Autodesk Fusion 360 part; units mm, degrees
(part 2 of 3)
extrude "Extrude4'''''''''" add sketch "Sketch4 (10)" along normal blind 20 separate body contours L0 L1 L2 L3 in plane through (0, 0, 580) normal (0, 0, 1) makes body 111 in component "02_VisionStation (1)"
sketch "Sketch5 (9)" plane through (0, 0, 0) normal (0, 0, 1) x (1, 0, 0) in component "02_VisionStation (1)"
  line L0 (965, 160, 540) -> (1015, 160, 540)
  line L1 (1015, 160, 540) -> (1015, 240, 540)
  line L2 (1015, 240, 540) -> (965, 240, 540)
  line L3 (965, 240, 540) -> (965, 160, 540)
extrude "Extrude5''''''''" add sketch "Sketch5 (9)" along normal blind 40 separate body contours L0 L1 L2 L3 in plane through (0, 0, 540) normal (0, 0, 1) makes body 112 in component "02_VisionStation (1)"
sketch "Sketch6 (9)" plane through (0, 0, 0) normal (0, 0, 1) x (1, 0, 0) in component "02_VisionStation (1)"
  circle A0 through (1002, 200, 520) (984, 210.3923, 520) (984, 189.6077, 520)
extrude "Extrude6''''''''" add sketch "Sketch6 (9)" along normal blind 20 separate body contours A0 in plane through (0, 0, 520) normal (0, 0, 1) makes body 113 in component "02_VisionStation (1)"
sketch "Sketch7 (9)" plane through (0, 0, 0) normal (0, 0, 1) x (1, 0, 0) in component "02_VisionStation (1)"
  line L0 (940, 180, 490) -> (1040, 180, 490)
  line L1 (1040, 180, 490) -> (1040, 220, 490)
  line L2 (1040, 220, 490) -> (940, 220, 490)
  line L3 (940, 220, 490) -> (940, 180, 490)
extrude "Extrude7''''''''" add sketch "Sketch7 (9)" along normal blind 25 separate body contours L0 L1 L2 L3 in plane through (0, 0, 490) normal (0, 0, 1) makes body 114 in component "02_VisionStation (1)"
sketch "Sketch8 (9)" plane through (0, 0, 0) normal (0, 0, 1) x (1, 0, 0) in component "02_VisionStation (1)"
  circle A0 through (972, 195, 480) (961.5, 201.0622, 480) (961.5, 188.9378, 480)
extrude "Extrude8''''''''" add sketch "Sketch8 (9)" along normal blind 10 separate body contours A0 in plane through (0, 0, 480) normal (0, 0, 1) makes body 115 in component "02_VisionStation (1)"
sketch "Sketch9 (9)" plane through (0, 0, 0) normal (0, 0, 1) x (1, 0, 0) in component "02_VisionStation (1)"
  circle A0 through (1022, 195, 480) (1011.5, 201.0622, 480) (1011.5, 188.9378, 480)
extrude "Extrude9''''''''" add sketch "Sketch9 (9)" along normal blind 10 separate body contours A0 in plane through (0, 0, 480) normal (0, 0, 1) makes body 116 in component "02_VisionStation (1)"
sketch "Sketch10 (9)" plane through (0, 0, 0) normal (0, 0, 1) x (1, 0, 0) in component "02_VisionStation (1)"
  circle A0 through (1025, 200, 530) (972.5, 230.3109, 530) (972.5, 169.6891, 530)
extrude "Extrude10''''''''" add sketch "Sketch10 (9)" along normal blind 5 separate body contours A0 in plane through (0, 0, 530) normal (0, 0, 1) makes body 117 in component "02_VisionStation (1)"
sketch "Sketch1 (12)" plane through (0, 0, 0) normal (0, 0, 1) x (1, 0, 0) in component "03_RobotBase (1)"
  line L0 (-200, -200) -> (200, -200)
  line L1 (200, -200) -> (200, 200)
  line L2 (200, 200) -> (-200, 200)
  line L3 (-200, 200) -> (-200, -200)
extrude "Extrude1'''''''''''" add sketch "Sketch1 (12)" along normal blind 30 separate body makes body 118 in component "03_RobotBase (1)"
sketch "Sketch2 (12)" plane through (0, 0, 0) normal (0, 0, 1) x (1, 0, 0) in component "03_RobotBase (1)"
  circle A0 through (150, 0, 30) (-75, 129.9038, 30) (-75, -129.9038, 30)
extrude "Extrude2'''''''''''" add sketch "Sketch2 (12)" along normal blind 100 separate body contours A0 in plane through (0, 0, 30) normal (0, 0, 1) makes body 119 in component "03_RobotBase (1)"
sketch "Sketch3 (11)" plane through (0, 0, 0) normal (0, 0, 1) x (1, 0, 0) in component "03_RobotBase (1)"
  circle A0 through (120, 0, 130) (-60, 103.923, 130) (-60, -103.923, 130)
extrude "Extrude3''''''''''" add sketch "Sketch3 (11)" along normal blind 20 separate body contours A0 in plane through (0, 0, 130) normal (0, 0, 1) makes body 120 in component "03_RobotBase (1)"
sketch "Sketch4 (11)" plane through (0, 0, 0) normal (0, 0, 1) x (1, 0, 0) in component "03_RobotBase (1)"
  line L0 (80, -40, 50) -> (136, -40, 50)
  line L1 (136, -40, 50) -> (136, 16, 50)
  line L2 (136, 16, 50) -> (80, 16, 50)
  line L3 (80, 16, 50) -> (80, -40, 50)
extrude "Extrude4''''''''''" add sketch "Sketch4 (11)" along normal blind 76 separate body contours L0 L1 L2 L3 in plane through (0, 0, 50) normal (0, 0, 1) makes body 121 in component "03_RobotBase (1)"
sketch "Sketch1 (13)" plane through (0, 0, 0) normal (0, 0, 1) x (1, 0, 0) in component "04_RobotArm (1)"
  circle A0 through (80, 0, 150) (-40, 69.282, 150) (-40, -69.282, 150)
extrude "Extrude1''''''''''''" add sketch "Sketch1 (13)" along normal blind 40 separate body contours A0 in plane through (0, 0, 150) normal (0, 0, 1) makes body 122 in component "04_RobotArm (1)"
sketch "Sketch2 (13)" plane through (0, 0, 0) normal (0, 0, 1) x (1, 0, 0) in component "04_RobotArm (1)"
  line L0 (-45, 50, 120) -> (11, 50, 120)
  line L1 (11, 50, 120) -> (11, 106, 120)
  line L2 (11, 106, 120) -> (-45, 106, 120)
  line L3 (-45, 106, 120) -> (-45, 50, 120)
extrude "Extrude2''''''''''''" add sketch "Sketch2 (13)" along normal blind 76 separate body contours L0 L1 L2 L3 in plane through (0, 0, 120) normal (0, 0, 1) makes body 123 in component "04_RobotArm (1)"
sketch "Sketch3 (12)" plane through (0, 0, 0) normal (0, 0, 1) x (1, 0, 0) in component "04_RobotArm (1)"
  line L0 (-20, -20, 190) -> (20, -20, 190)
  line L1 (20, -20, 190) -> (20, 20, 190)
  line L2 (20, 20, 190) -> (-20, 20, 190)
  line L3 (-20, 20, 190) -> (-20, -20, 190)
extrude "Extrude3'''''''''''" add sketch "Sketch3 (12)" along normal blind 400 separate body contours L0 L1 L2 L3 in plane through (0, 0, 190) normal (0, 0, 1) makes body 124 in component "04_RobotArm (1)"
sketch "Sketch4 (12)" plane through (0, 0, 0) normal (0, 0, 1) x (1, 0, 0) in component "04_RobotArm (1)"
  line L0 (-25, -25, 250) -> (25, -25, 250)
  line L1 (25, -25, 250) -> (25, 25, 250)
  line L2 (25, 25, 250) -> (-25, 25, 250)
  line L3 (-25, 25, 250) -> (-25, -25, 250)
extrude "Extrude4'''''''''''" add sketch "Sketch4 (12)" along normal blind 5 separate body contours L0 L1 L2 L3 in plane through (0, 0, 250) normal (0, 0, 1) makes body 125 in component "04_RobotArm (1)"
sketch "Sketch5 (10)" plane through (0, 0, 0) normal (0, 0, 1) x (1, 0, 0) in component "04_RobotArm (1)"
  line L0 (-25, -25, 350) -> (25, -25, 350)
  line L1 (25, -25, 350) -> (25, 25, 350)
  line L2 (25, 25, 350) -> (-25, 25, 350)
  line L3 (-25, 25, 350) -> (-25, -25, 350)
extrude "Extrude5'''''''''" add sketch "Sketch5 (10)" along normal blind 5 separate body contours L0 L1 L2 L3 in plane through (0, 0, 350) normal (0, 0, 1) makes body 126 in component "04_RobotArm (1)"
sketch "Sketch6 (10)" plane through (0, 0, 0) normal (0, 0, 1) x (1, 0, 0) in component "04_RobotArm (1)"
  line L0 (-25, -25, 450) -> (25, -25, 450)
  line L1 (25, -25, 450) -> (25, 25, 450)
  line L2 (25, 25, 450) -> (-25, 25, 450)
  line L3 (-25, 25, 450) -> (-25, -25, 450)
extrude "Extrude6'''''''''" add sketch "Sketch6 (10)" along normal blind 5 separate body contours L0 L1 L2 L3 in plane through (0, 0, 450) normal (0, 0, 1) makes body 127 in component "04_RobotArm (1)"
sketch "Sketch7 (10)" plane through (0, 0, 0) normal (0, 0, 1) x (1, 0, 0) in component "04_RobotArm (1)"
  circle A0 through (60, 0, 590) (-30, 51.9615, 590) (-30, -51.9615, 590)
extrude "Extrude7'''''''''" add sketch "Sketch7 (10)" along normal blind 40 separate body contours A0 in plane through (0, 0, 590) normal (0, 0, 1) makes body 128 in component "04_RobotArm (1)"
sketch "Sketch8 (10)" plane through (0, 0, 0) normal (0, 0, 1) x (1, 0, 0) in component "04_RobotArm (1)"
  line L0 (50, -30, 570) -> (106, -30, 570)
  line L1 (106, -30, 570) -> (106, 26, 570)
  line L2 (106, 26, 570) -> (50, 26, 570)
  line L3 (50, 26, 570) -> (50, -30, 570)
extrude "Extrude8'''''''''" add sketch "Sketch8 (10)" along normal blind 76 separate body contours L0 L1 L2 L3 in plane through (0, 0, 570) normal (0, 0, 1) makes body 129 in component "04_RobotArm (1)"
sketch "Sketch9 (10)" plane through (0, 0, 0) normal (0, 0, 1) x (1, 0, 0) in component "04_RobotArm (1)"
  line L0 (-20, -20, 630) -> (20, -20, 630)
  line L1 (20, -20, 630) -> (20, 20, 630)
  line L2 (20, 20, 630) -> (-20, 20, 630)
  line L3 (-20, 20, 630) -> (-20, -20, 630)
extrude "Extrude9'''''''''" add sketch "Sketch9 (10)" along normal blind 350 separate body contours L0 L1 L2 L3 in plane through (0, 0, 630) normal (0, 0, 1) makes body 130 in component "04_RobotArm (1)"
sketch "Sketch10 (10)" plane through (0, 0, 0) normal (0, 0, 1) x (1, 0, 0) in component "04_RobotArm (1)"
  circle A0 through (50, 0, 980) (-25, 43.3013, 980) (-25, -43.3013, 980)
extrude "Extrude10'''''''''" add sketch "Sketch10 (10)" along normal blind 30 separate body contours A0 in plane through (0, 0, 980) normal (0, 0, 1) makes body 131 in component "04_RobotArm (1)"
sketch "Sketch11 (5)" plane through (0, 0, 0) normal (0, 0, 1) x (1, 0, 0) in component "04_RobotArm (1)"
  line L0 (30, -20, 960) -> (70, -20, 960)
  line L1 (70, -20, 960) -> (70, 20, 960)
  line L2 (70, 20, 960) -> (30, 20, 960)
  line L3 (30, 20, 960) -> (30, -20, 960)
extrude "Extrude11''''" add sketch "Sketch11 (5)" along normal blind 50 separate body contours L0 L1 L2 L3 in plane through (0, 0, 960) normal (0, 0, 1) makes body 132 in component "04_RobotArm (1)"
sketch "Sketch12 (4)" plane through (0, 0, 0) normal (0, 0, 1) x (1, 0, 0) in component "04_RobotArm (1)"
  circle A0 through (-15, 30, 130) (-37.5, 42.9904, 130) (-37.5, 17.0096, 130)
extrude "Extrude12'''" add sketch "Sketch12 (4)" along normal blind 15 separate body contours A0 in plane through (0, 0, 130) normal (0, 0, 1) makes body 133 in component "04_RobotArm (1)"
sketch "Sketch13 (4)" plane through (0, 0, 0) normal (0, 0, 1) x (1, 0, 0) in component "04_RobotArm (1)"
  circle A0 through (-15, 30, 570) (-37.5, 42.9904, 570) (-37.5, 17.0096, 570)
extrude "Extrude13'''" add sketch "Sketch13 (4)" along normal blind 15 separate body contours A0 in plane through (0, 0, 570) normal (0, 0, 1) makes body 134 in component "04_RobotArm (1)"
sketch "Sketch14 (4)" plane through (0, 0, 0) normal (0, 0, 1) x (1, 0, 0) in component "04_RobotArm (1)"
  circle A0 through (-15, 30, 960) (-37.5, 42.9904, 960) (-37.5, 17.0096, 960)
extrude "Extrude14'''" add sketch "Sketch14 (4)" along normal blind 15 separate body contours A0 in plane through (0, 0, 960) normal (0, 0, 1) makes body 135 in component "04_RobotArm (1)"
sketch "Sketch1 (14)" plane through (0, 0, 0) normal (0, 0, 1) x (1, 0, 0) in component "05_Gripper (1)"
  line L0 (-50, -30) -> (50, -30)
  line L1 (50, -30) -> (50, 30)
  line L2 (50, 30) -> (-50, 30)
  line L3 (-50, 30) -> (-50, -30)
extrude "Extrude1'''''''''''''" add sketch "Sketch1 (14)" along normal blind 60 separate body makes body 136 in component "05_Gripper (1)"
sketch "Sketch2 (14)" plane through (0, 0, 0) normal (0, 0, 1) x (1, 0, 0) in component "05_Gripper (1)"
  line L0 (-75, -30) -> (-50, -30)
  line L1 (-50, -30) -> (-50, 30)
  line L2 (-50, 30) -> (-75, 30)
  line L3 (-75, 30) -> (-75, -30)
extrude "Extrude2'''''''''''''" add sketch "Sketch2 (14)" along normal blind 50 separate body makes body 137 in component "05_Gripper (1)"
sketch "Sketch3 (13)" plane through (0, 0, 0) normal (0, 0, 1) x (1, 0, 0) in component "05_Gripper (1)"
  line L0 (50, -30) -> (75, -30)
  line L1 (75, -30) -> (75, 30)
  line L2 (75, 30) -> (50, 30)
  line L3 (50, 30) -> (50, -30)
extrude "Extrude3''''''''''''" add sketch "Sketch3 (13)" along normal blind 50 separate body makes body 138 in component "05_Gripper (1)"
sketch "Sketch4 (13)" plane through (0, 0, 0) normal (0, 0, 1) x (1, 0, 0) in component "05_Gripper (1)"
  line L0 (-50, -25, 10) -> (50, -25, 10)
  line L1 (50, -25, 10) -> (50, -21, 10)
  line L2 (50, -21, 10) -> (-50, -21, 10)
  line L3 (-50, -21, 10) -> (-50, -25, 10)
extrude "Extrude4''''''''''''" add sketch "Sketch4 (13)" along normal blind 30 separate body contours L0 L1 L2 L3 in plane through (0, 0, 10) normal (0, 0, 1) makes body 139 in component "05_Gripper (1)"
sketch "Sketch5 (11)" plane through (0, 0, 0) normal (0, 0, 1) x (1, 0, 0) in component "05_Gripper (1)"
  line L0 (-50, 25, 10) -> (50, 25, 10)
  line L1 (50, 25, 10) -> (50, 29, 10)
  line L2 (50, 29, 10) -> (-50, 29, 10)
  line L3 (-50, 29, 10) -> (-50, 25, 10)
extrude "Extrude5''''''''''" add sketch "Sketch5 (11)" along normal blind 30 separate body contours L0 L1 L2 L3 in plane through (0, 0, 10) normal (0, 0, 1) makes body 140 in component "05_Gripper (1)"
sketch "Sketch6 (11)" plane through (0, 0, 0) normal (0, 0, 1) x (1, 0, 0) in component "05_Gripper (1)"
  circle A0 through (25, 0, 60) (-12.5, 21.6506, 60) (-12.5, -21.6506, 60)
extrude "Extrude6''''''''''" add sketch "Sketch6 (11)" along normal blind 80 separate body contours A0 in plane through (0, 0, 60) normal (0, 0, 1) makes body 141 in component "05_Gripper (1)"
sketch "Sketch7 (11)" plane through (0, 0, 0) normal (0, 0, 1) x (1, 0, 0) in component "05_Gripper (1)"
  circle A0 through (-16, 0, 140) (-22, 3.4641, 140) (-22, -3.4641, 140)
extrude "Extrude7''''''''''" add sketch "Sketch7 (11)" along normal blind 30 separate body contours A0 in plane through (0, 0, 140) normal (0, 0, 1) makes body 142 in component "05_Gripper (1)"
sketch "Sketch8 (11)" plane through (0, 0, 0) normal (0, 0, 1) x (1, 0, 0) in component "05_Gripper (1)"
  circle A0 through (24, 0, 140) (18, 3.4641, 140) (18, -3.4641, 140)
extrude "Extrude8''''''''''" add sketch "Sketch8 (11)" along normal blind 30 separate body contours A0 in plane through (0, 0, 140) normal (0, 0, 1) makes body 143 in component "05_Gripper (1)"
sketch "Sketch9 (11)" plane through (0, 0, 0) normal (0, 0, 1) x (1, 0, 0) in component "05_Gripper (1)"
  circle A0 through (30, 0, -20) (-15, 25.9808, -20) (-15, -25.9808, -20)
extrude "Extrude9''''''''''" add sketch "Sketch9 (11)" along normal blind 20 separate body contours A0 in plane through (0, 0, -20) normal (0, 0, 1) makes body 144 in component "05_Gripper (1)"
sketch "Sketch10 (11)" plane through (0, 0, 0) normal (0, 0, 1) x (1, 0, 0) in component "05_Gripper (1)"
  line L0 (-10, -5, -5) -> (10, -5, -5)
  line L1 (10, -5, -5) -> (10, 5, -5)
  line L2 (10, 5, -5) -> (-10, 5, -5)
  line L3 (-10, 5, -5) -> (-10, -5, -5)
extrude "Extrude10''''''''''" add sketch "Sketch10 (11)" along normal blind 3 separate body contours L0 L1 L2 L3 in plane through (0, 0, -5) normal (0, 0, 1) makes body 145 in component "05_Gripper (1)"
sketch "Sketch11 (6)" plane through (0, 0, 0) normal (0, 0, 1) x (1, 0, 0) in component "05_Gripper (1)"
  line L0 (-35, 35, 20) -> (35, 35, 20)
  line L1 (35, 35, 20) -> (35, 65, 20)
  line L2 (35, 65, 20) -> (-35, 65, 20)
  line L3 (-35, 65, 20) -> (-35, 35, 20)
extrude "Extrude11'''''" add sketch "Sketch11 (6)" along normal blind 40 separate body contours L0 L1 L2 L3 in plane through (0, 0, 20) normal (0, 0, 1) makes body 146 in component "05_Gripper (1)"
sketch "Sketch1 (15)" plane through (0, 0, 0) normal (0, 0, 1) x (1, 0, 0) in component "06_SortingBins (1)"
  line L0 (396.8309, 88.1111) -> (636.8309, 88.1111)
  line L1 (636.8309, 88.1111) -> (636.8309, 288.1111)
  line L2 (636.8309, 288.1111) -> (396.8309, 288.1111)
  line L3 (396.8309, 288.1111) -> (396.8309, 88.1111)
extrude "Extrude1''''''''''''''" add sketch "Sketch1 (15)" along normal blind 250 separate body makes body 147 in component "06_SortingBins (1)"
sketch "Sketch2 (15)" plane through (0, 0, 0) normal (0, 0, 1) x (1, 0, 0) in component "06_SortingBins (1)"
  line L0 (456.8309, 83.1111, 80) -> (576.8309, 83.1111, 80)
  line L1 (576.8309, 83.1111, 80) -> (576.8309, 86.1111, 80)
  line L2 (576.8309, 86.1111, 80) -> (456.8309, 86.1111, 80)
  line L3 (456.8309, 86.1111, 80) -> (456.8309, 83.1111, 80)
extrude "Extrude2''''''''''''''" add sketch "Sketch2 (15)" along normal blind 60 separate body contours L0 L1 L2 L3 in plane through (0, 0, 80) normal (0, 0, 1) makes body 148 in component "06_SortingBins (1)"
sketch "Sketch3 (14)" plane through (0, 0, 0) normal (0, 0, 1) x (1, 0, 0) in component "06_SortingBins (1)"
  line L0 (396.8309, 88.1111, -15) -> (636.8309, 88.1111, -15)
  line L1 (636.8309, 88.1111, -15) -> (636.8309, 288.1111, -15)
  line L2 (636.8309, 288.1111, -15) -> (396.8309, 288.1111, -15)
  line L3 (396.8309, 288.1111, -15) -> (396.8309, 88.1111, -15)
extrude "Extrude3'''''''''''''" add sketch "Sketch3 (14)" along normal blind 15 separate body contours L0 L1 L2 L3 in plane through (0, 0, -15) normal (0, 0, 1) makes body 149 in component "06_SortingBins (1)"
sketch "Sketch4 (14)" plane through (0, 0, 0) normal (0, 0, 1) x (1, 0, 0) in component "06_SortingBins (1)"
  line L0 (280.0555, 277.4329) -> (520.0555, 277.4329)
  line L1 (520.0555, 277.4329) -> (520.0555, 477.4329)
  line L2 (520.0555, 477.4329) -> (280.0555, 477.4329)
  line L3 (280.0555, 477.4329) -> (280.0555, 277.4329)
extrude "Extrude4'''''''''''''" add sketch "Sketch4 (14)" along normal blind 250 separate body makes body 150 in component "06_SortingBins (1)"
sketch "Sketch5 (12)" plane through (0, 0, 0) normal (0, 0, 1) x (1, 0, 0) in component "06_SortingBins (1)"
  line L0 (340.0555, 272.4329, 80) -> (460.0555, 272.4329, 80)
  line L1 (460.0555, 272.4329, 80) -> (460.0555, 275.4329, 80)
  line L2 (460.0555, 275.4329, 80) -> (340.0555, 275.4329, 80)
  line L3 (340.0555, 275.4329, 80) -> (340.0555, 272.4329, 80)
extrude "Extrude5'''''''''''" add sketch "Sketch5 (12)" along normal blind 60 separate body contours L0 L1 L2 L3 in plane through (0, 0, 80) normal (0, 0, 1) makes body 151 in component "06_SortingBins (1)"
sketch "Sketch6 (12)" plane through (0, 0, 0) normal (0, 0, 1) x (1, 0, 0) in component "06_SortingBins (1)"
  line L0 (280.0555, 277.4329, -15) -> (520.0555, 277.4329, -15)
  line L1 (520.0555, 277.4329, -15) -> (520.0555, 477.4329, -15)
  line L2 (520.0555, 477.4329, -15) -> (280.0555, 477.4329, -15)
  line L3 (280.0555, 477.4329, -15) -> (280.0555, 277.4329, -15)
extrude "Extrude6'''''''''''" add sketch "Sketch6 (12)" along normal blind 15 separate body contours L0 L1 L2 L3 in plane through (0, 0, -15) normal (0, 0, 1) makes body 152 in component "06_SortingBins (1)"
sketch "Sketch7 (12)" plane through (0, 0, 0) normal (0, 0, 1) x (1, 0, 0) in component "06_SortingBins (1)"
  line L0 (97.8439, 405.0189) -> (337.8439, 405.0189)
  line L1 (337.8439, 405.0189) -> (337.8439, 605.0189)
  line L2 (337.8439, 605.0189) -> (97.8439, 605.0189)
  line L3 (97.8439, 605.0189) -> (97.8439, 405.0189)
extrude "Extrude7'''''''''''" add sketch "Sketch7 (12)" along normal blind 250 separate body makes body 153 in component "06_SortingBins (1)"
sketch "Sketch8 (12)" plane through (0, 0, 0) normal (0, 0, 1) x (1, 0, 0) in component "06_SortingBins (1)"
  line L0 (157.8439, 400.0189, 80) -> (277.8439, 400.0189, 80)
  line L1 (277.8439, 400.0189, 80) -> (277.8439, 403.0189, 80)
  line L2 (277.8439, 403.0189, 80) -> (157.8439, 403.0189, 80)
  line L3 (157.8439, 403.0189, 80) -> (157.8439, 400.0189, 80)
extrude "Extrude8'''''''''''" add sketch "Sketch8 (12)" along normal blind 60 separate body contours L0 L1 L2 L3 in plane through (0, 0, 80) normal (0, 0, 1) makes body 154 in component "06_SortingBins (1)"
sketch "Sketch9 (12)" plane through (0, 0, 0) normal (0, 0, 1) x (1, 0, 0) in component "06_SortingBins (1)"
  line L0 (97.8439, 405.0189, -15) -> (337.8439, 405.0189, -15)
  line L1 (337.8439, 405.0189, -15) -> (337.8439, 605.0189, -15)
  line L2 (337.8439, 605.0189, -15) -> (97.8439, 605.0189, -15)
  line L3 (97.8439, 605.0189, -15) -> (97.8439, 405.0189, -15)
extrude "Extrude9'''''''''''" add sketch "Sketch9 (12)" along normal blind 15 separate body contours L0 L1 L2 L3 in plane through (0, 0, -15) normal (0, 0, 1) makes body 155 in component "06_SortingBins (1)"
sketch "Sketch10 (12)" plane through (0, 0, 0) normal (0, 0, 1) x (1, 0, 0) in component "06_SortingBins (1)"
  line L0 (-120, 450) -> (120, 450)
  line L1 (120, 450) -> (120, 650)
  line L2 (120, 650) -> (-120, 650)
  line L3 (-120, 650) -> (-120, 450)
extrude "Extrude10'''''''''''" add sketch "Sketch10 (12)" along normal blind 250 separate body makes body 156 in component "06_SortingBins (1)"
sketch "Sketch11 (7)" plane through (0, 0, 0) normal (0, 0, 1) x (1, 0, 0) in component "06_SortingBins (1)"
  line L0 (-60, 445, 80) -> (60, 445, 80)
  line L1 (60, 445, 80) -> (60, 448, 80)
  line L2 (60, 448, 80) -> (-60, 448, 80)
  line L3 (-60, 448, 80) -> (-60, 445, 80)
extrude "Extrude11''''''" add sketch "Sketch11 (7)" along normal blind 60 separate body contours L0 L1 L2 L3 in plane through (0, 0, 80) normal (0, 0, 1) makes body 157 in component "06_SortingBins (1)"
sketch "Sketch12 (5)" plane through (0, 0, 0) normal (0, 0, 1) x (1, 0, 0) in component "06_SortingBins (1)"
  line L0 (-120, 450, -15) -> (120, 450, -15)
  line L1 (120, 450, -15) -> (120, 650, -15)
  line L2 (120, 650, -15) -> (-120, 650, -15)
  line L3 (-120, 650, -15) -> (-120, 450, -15)
extrude "Extrude12''''" add sketch "Sketch12 (5)" along normal blind 15 separate body contours L0 L1 L2 L3 in plane through (0, 0, -15) normal (0, 0, 1) makes body 158 in component "06_SortingBins (1)"
sketch "Sketch13 (5)" plane through (0, 0, 0) normal (0, 0, 1) x (1, 0, 0) in component "06_SortingBins (1)"
  line L0 (-337.8439, 405.0189) -> (-97.8439, 405.0189)
  line L1 (-97.8439, 405.0189) -> (-97.8439, 605.0189)
  line L2 (-97.8439, 605.0189) -> (-337.8439, 605.0189)
  line L3 (-337.8439, 605.0189) -> (-337.8439, 405.0189)
extrude "Extrude13''''" add sketch "Sketch13 (5)" along normal blind 250 separate body makes body 159 in component "06_SortingBins (1)"
sketch "Sketch14 (5)" plane through (0, 0, 0) normal (0, 0, 1) x (1, 0, 0) in component "06_SortingBins (1)"
  line L0 (-277.8439, 400.0189, 80) -> (-157.8439, 400.0189, 80)
  line L1 (-157.8439, 400.0189, 80) -> (-157.8439, 403.0189, 80)
  line L2 (-157.8439, 403.0189, 80) -> (-277.8439, 403.0189, 80)
  line L3 (-277.8439, 403.0189, 80) -> (-277.8439, 400.0189, 80)
extrude "Extrude14''''" add sketch "Sketch14 (5)" along normal blind 60 separate body contours L0 L1 L2 L3 in plane through (0, 0, 80) normal (0, 0, 1) makes body 160 in component "06_SortingBins (1)"
sketch "Sketch15 (3)" plane through (0, 0, 0) normal (0, 0, 1) x (1, 0, 0) in component "06_SortingBins (1)"
  line L0 (-337.8439, 405.0189, -15) -> (-97.8439, 405.0189, -15)
  line L1 (-97.8439, 405.0189, -15) -> (-97.8439, 605.0189, -15)
  line L2 (-97.8439, 605.0189, -15) -> (-337.8439, 605.0189, -15)
  line L3 (-337.8439, 605.0189, -15) -> (-337.8439, 405.0189, -15)
extrude "Extrude15''" add sketch "Sketch15 (3)" along normal blind 15 separate body contours L0 L1 L2 L3 in plane through (0, 0, -15) normal (0, 0, 1) makes body 161 in component "06_SortingBins (1)"
sketch "Sketch16 (2)" plane through (0, 0, 0) normal (0, 0, 1) x (1, 0, 0) in component "06_SortingBins (1)"
  line L0 (-520.0555, 277.4329) -> (-280.0555, 277.4329)
  line L1 (-280.0555, 277.4329) -> (-280.0555, 477.4329)
  line L2 (-280.0555, 477.4329) -> (-520.0555, 477.4329)
  line L3 (-520.0555, 477.4329) -> (-520.0555, 277.4329)
extrude "Extrude16'" add sketch "Sketch16 (2)" along normal blind 250 separate body makes body 162 in component "06_SortingBins (1)"
sketch "Sketch17 (2)" plane through (0, 0, 0) normal (0, 0, 1) x (1, 0, 0) in component "06_SortingBins (1)"
  line L0 (-460.0555, 272.4329, 80) -> (-340.0555, 272.4329, 80)
  line L1 (-340.0555, 272.4329, 80) -> (-340.0555, 275.4329, 80)
  line L2 (-340.0555, 275.4329, 80) -> (-460.0555, 275.4329, 80)
  line L3 (-460.0555, 275.4329, 80) -> (-460.0555, 272.4329, 80)
extrude "Extrude17'" add sketch "Sketch17 (2)" along normal blind 60 separate body contours L0 L1 L2 L3 in plane through (0, 0, 80) normal (0, 0, 1) makes body 163 in component "06_SortingBins (1)"
sketch "Sketch18 (2)" plane through (0, 0, 0) normal (0, 0, 1) x (1, 0, 0) in component "06_SortingBins (1)"
  line L0 (-520.0555, 277.4329, -15) -> (-280.0555, 277.4329, -15)
  line L1 (-280.0555, 277.4329, -15) -> (-280.0555, 477.4329, -15)
  line L2 (-280.0555, 477.4329, -15) -> (-520.0555, 477.4329, -15)
  line L3 (-520.0555, 477.4329, -15) -> (-520.0555, 277.4329, -15)
extrude "Extrude18'" add sketch "Sketch18 (2)" along normal blind 15 separate body contours L0 L1 L2 L3 in plane through (0, 0, -15) normal (0, 0, 1) makes body 164 in component "06_SortingBins (1)"
sketch "Sketch19 (2)" plane through (0, 0, 0) normal (0, 0, 1) x (1, 0, 0) in component "06_SortingBins (1)"
  line L0 (-636.8309, 88.1111) -> (-396.8309, 88.1111)
  line L1 (-396.8309, 88.1111) -> (-396.8309, 288.1111)
  line L2 (-396.8309, 288.1111) -> (-636.8309, 288.1111)
  line L3 (-636.8309, 288.1111) -> (-636.8309, 88.1111)
extrude "Extrude19'" add sketch "Sketch19 (2)" along normal blind 250 separate body makes body 165 in component "06_SortingBins (1)"
sketch "Sketch20 (2)" plane through (0, 0, 0) normal (0, 0, 1) x (1, 0, 0) in component "06_SortingBins (1)"
  line L0 (-576.8309, 83.1111, 80) -> (-456.8309, 83.1111, 80)
  line L1 (-456.8309, 83.1111, 80) -> (-456.8309, 86.1111, 80)
  line L2 (-456.8309, 86.1111, 80) -> (-576.8309, 86.1111, 80)
  line L3 (-576.8309, 86.1111, 80) -> (-576.8309, 83.1111, 80)
extrude "Extrude20'" add sketch "Sketch20 (2)" along normal blind 60 separate body contours L0 L1 L2 L3 in plane through (0, 0, 80) normal (0, 0, 1) makes body 166 in component "06_SortingBins (1)"
sketch "Sketch21 (2)" plane through (0, 0, 0) normal (0, 0, 1) x (1, 0, 0) in component "06_SortingBins (1)"
  line L0 (-636.8309, 88.1111, -15) -> (-396.8309, 88.1111, -15)
  line L1 (-396.8309, 88.1111, -15) -> (-396.8309, 288.1111, -15)
  line L2 (-396.8309, 288.1111, -15) -> (-636.8309, 288.1111, -15)
  line L3 (-636.8309, 288.1111, -15) -> (-636.8309, 88.1111, -15)
extrude "Extrude21'" add sketch "Sketch21 (2)" along normal blind 15 separate body contours L0 L1 L2 L3 in plane through (0, 0, -15) normal (0, 0, 1) makes body 167 in component "06_SortingBins (1)"
sketch "Sketch1 (16)" plane through (0, 0, 0) normal (0, 0, 1) x (1, 0, 0) in component "07_ComputeCabinet (1)"
  line L0 (0, 0) -> (500, 0)
  line L1 (500, 0) -> (500, 300)
  line L2 (500, 300) -> (0, 300)
  line L3 (0, 300) -> (0, 0)
extrude "Extrude1'''''''''''''''" add sketch "Sketch1 (16)" along normal blind 700 separate body makes body 168 in component "07_ComputeCabinet (1)"
sketch "Sketch2 (16)" plane through (0, 0, 0) normal (0, 0, 1) x (1, 0, 0) in component "07_ComputeCabinet (1)"
  line L0 (0, -5, 50) -> (500, -5, 50)
  line L1 (500, -5, 50) -> (500, 0, 50)
  line L2 (500, 0, 50) -> (0, 0, 50)
  line L3 (0, 0, 50) -> (0, -5, 50)
extrude "Extrude2'''''''''''''''" add sketch "Sketch2 (16)" along normal blind 600 separate body contours L0 L1 L2 L3 in plane through (0, 0, 50) normal (0, 0, 1) makes body 169 in component "07_ComputeCabinet (1)"
sketch "Sketch3 (15)" plane through (0, 0, 0) normal (0, 0, 1) x (1, 0, 0) in component "07_ComputeCabinet (1)"
  line L0 (30, 50, 120) -> (470, 50, 120)
  line L1 (470, 50, 120) -> (470, 54, 120)
  line L2 (470, 54, 120) -> (30, 54, 120)
  line L3 (30, 54, 120) -> (30, 50, 120)
extrude "Extrude3''''''''''''''" add sketch "Sketch3 (15)" along normal blind 15 separate body contours L0 L1 L2 L3 in plane through (0, 0, 120) normal (0, 0, 1) makes body 170 in component "07_ComputeCabinet (1)"
sketch "Sketch4 (15)" plane through (0, 0, 0) normal (0, 0, 1) x (1, 0, 0) in component "07_ComputeCabinet (1)"
  line L0 (30, 50, 300) -> (470, 50, 300)
  line L1 (470, 50, 300) -> (470, 54, 300)
  line L2 (470, 54, 300) -> (30, 54, 300)
  line L3 (30, 54, 300) -> (30, 50, 300)
extrude "Extrude4''''''''''''''" add sketch "Sketch4 (15)" along normal blind 15 separate body contours L0 L1 L2 L3 in plane through (0, 0, 300) normal (0, 0, 1) makes body 171 in component "07_ComputeCabinet (1)"
sketch "Sketch5 (13)" plane through (0, 0, 0) normal (0, 0, 1) x (1, 0, 0) in component "07_ComputeCabinet (1)"
  line L0 (30, 50, 500) -> (470, 50, 500)
  line L1 (470, 50, 500) -> (470, 54, 500)
  line L2 (470, 54, 500) -> (30, 54, 500)
  line L3 (30, 54, 500) -> (30, 50, 500)
extrude "Extrude5''''''''''''" add sketch "Sketch5 (13)" along normal blind 15 separate body contours L0 L1 L2 L3 in plane through (0, 0, 500) normal (0, 0, 1) makes body 172 in component "07_ComputeCabinet (1)"
sketch "Sketch6 (13)" plane through (0, 0, 0) normal (0, 0, 1) x (1, 0, 0) in component "07_ComputeCabinet (1)"
  line L0 (40, 60, 140) -> (140, 60, 140)
  line L1 (140, 60, 140) -> (140, 140, 140)
  line L2 (140, 140, 140) -> (40, 140, 140)
  line L3 (40, 140, 140) -> (40, 60, 140)
extrude "Extrude6''''''''''''" add sketch "Sketch6 (13)" along normal blind 60 separate body contours L0 L1 L2 L3 in plane through (0, 0, 140) normal (0, 0, 1) makes body 173 in component "07_ComputeCabinet (1)"
sketch "Sketch7 (13)" plane through (0, 0, 0) normal (0, 0, 1) x (1, 0, 0) in component "07_ComputeCabinet (1)"
  circle A0 through (120, 100, 200) (75, 125.9808, 200) (75, 74.0192, 200)
extrude "Extrude7''''''''''''" add sketch "Sketch7 (13)" along normal blind 10 separate body contours A0 in plane through (0, 0, 200) normal (0, 0, 1) makes body 174 in component "07_ComputeCabinet (1)"
sketch "Sketch8 (13)" plane through (0, 0, 0) normal (0, 0, 1) x (1, 0, 0) in component "07_ComputeCabinet (1)"
  line L0 (180, 60, 140) -> (240, 60, 140)
  line L1 (240, 60, 140) -> (240, 100, 140)
  line L2 (240, 100, 140) -> (180, 100, 140)
  line L3 (180, 100, 140) -> (180, 60, 140)
extrude "Extrude8''''''''''''" add sketch "Sketch8 (13)" along normal blind 10 separate body contours L0 L1 L2 L3 in plane through (0, 0, 140) normal (0, 0, 1) makes body 175 in component "07_ComputeCabinet (1)"
sketch "Sketch9 (13)" plane through (0, 0, 0) normal (0, 0, 1) x (1, 0, 0) in component "07_ComputeCabinet (1)"
  line L0 (270, 60, 140) -> (350, 60, 140)
  line L1 (350, 60, 140) -> (350, 80, 140)
  line L2 (350, 80, 140) -> (270, 80, 140)
  line L3 (270, 80, 140) -> (270, 60, 140)
extrude "Extrude9''''''''''''" add sketch "Sketch9 (13)" along normal blind 4 separate body contours L0 L1 L2 L3 in plane through (0, 0, 140) normal (0, 0, 1) makes body 176 in component "07_ComputeCabinet (1)"
sketch "Sketch10 (13)" plane through (0, 0, 0) normal (0, 0, 1) x (1, 0, 0) in component "07_ComputeCabinet (1)"
  line L0 (40, 60, 320) -> (220, 60, 320)
  line L1 (220, 60, 320) -> (220, 160, 320)
  line L2 (220, 160, 320) -> (40, 160, 320)
  line L3 (40, 160, 320) -> (40, 60, 320)
extrude "Extrude10''''''''''''" add sketch "Sketch10 (13)" along normal blind 60 separate body contours L0 L1 L2 L3 in plane through (0, 0, 320) normal (0, 0, 1) makes body 177 in component "07_ComputeCabinet (1)"
sketch "Sketch11 (8)" plane through (0, 0, 0) normal (0, 0, 1) x (1, 0, 0) in component "07_ComputeCabinet (1)"
  line L0 (260, 60, 320) -> (440, 60, 320)
  line L1 (440, 60, 320) -> (440, 160, 320)
  line L2 (440, 160, 320) -> (260, 160, 320)
  line L3 (260, 160, 320) -> (260, 60, 320)
extrude "Extrude11'''''''" add sketch "Sketch11 (8)" along normal blind 60 separate body contours L0 L1 L2 L3 in plane through (0, 0, 320) normal (0, 0, 1) makes body 178 in component "07_ComputeCabinet (1)"
sketch "Sketch12 (6)" plane through (0, 0, 0) normal (0, 0, 1) x (1, 0, 0) in component "07_ComputeCabinet (1)"
  line L0 (40, 60, 520) -> (420, 60, 520)
  line L1 (420, 60, 520) -> (420, 200, 520)
  line L2 (420, 200, 520) -> (40, 200, 520)
  line L3 (40, 200, 520) -> (40, 60, 520)
extrude "Extrude12'''''" add sketch "Sketch12 (6)" along normal blind 100 separate body contours L0 L1 L2 L3 in plane through (0, 0, 520) normal (0, 0, 1) makes body 179 in component "07_ComputeCabinet (1)"
sketch "Sketch13 (6)" plane through (0, 0, 0) normal (0, 0, 1) x (1, 0, 0) in component "07_ComputeCabinet (1)"
  circle A0 through (80, -3, 550) (35, 22.9808, 550) (35, -28.9808, 550)
extrude "Extrude13'''''" add sketch "Sketch13 (6)" along normal blind 30 separate body contours A0 in plane through (0, 0, 550) normal (0, 0, 1) makes body 180 in component "07_ComputeCabinet (1)"
sketch "Sketch14 (6)" plane through (0, 0, 0) normal (0, 0, 1) x (1, 0, 0) in component "07_ComputeCabinet (1)"
  line L0 (360, 60, 140) -> (420, 60, 140)
  line L1 (420, 60, 140) -> (420, 100, 140)
  line L2 (420, 100, 140) -> (360, 100, 140)
  line L3 (360, 100, 140) -> (360, 60, 140)
extrude "Extrude14'''''" add sketch "Sketch14 (6)" along normal blind 40 separate body contours L0 L1 L2 L3 in plane through (0, 0, 140) normal (0, 0, 1) makes body 181 in component "07_ComputeCabinet (1)"
sketch "Sketch15 (4)" plane through (0, 0, 0) normal (0, 0, 1) x (1, 0, 0) in component "07_ComputeCabinet (1)"
  line L0 (180, 60, 220) -> (220, 60, 220)
  line L1 (220, 60, 220) -> (220, 85, 220)
  line L2 (220, 85, 220) -> (180, 85, 220)
  line L3 (180, 85, 220) -> (180, 60, 220)
extrude "Extrude15'''" add sketch "Sketch15 (4)" along normal blind 3 separate body contours L0 L1 L2 L3 in plane through (0, 0, 220) normal (0, 0, 1) makes body 182 in component "07_ComputeCabinet (1)"
sketch "Sketch1 (17)" plane through (0, 0, 0) normal (0, 0, 1) x (1, 0, 0) in component "08_PneumaticSystem (1)"
  line L0 (0, 0) -> (300, 0)
  line L1 (300, 0) -> (300, 200)
  line L2 (300, 200) -> (0, 200)
  line L3 (0, 200) -> (0, 0)
extrude "Extrude1''''''''''''''''" add sketch "Sketch1 (17)" along normal blind 350 separate body makes body 183 in component "08_PneumaticSystem (1)"
sketch "Sketch2 (17)" plane through (0, 0, 0) normal (0, 0, 1) x (1, 0, 0) in component "08_PneumaticSystem (1)"
  circle A0 through (230, 100, 350) (110, 169.282, 350) (110, 30.718, 350)
extrude "Extrude2''''''''''''''''" add sketch "Sketch2 (17)" along normal blind 200 separate body contours A0 in plane through (0, 0, 350) normal (0, 0, 1) makes body 184 in component "08_PneumaticSystem (1)"
sketch "Sketch3 (16)" plane through (0, 0, 0) normal (0, 0, 1) x (1, 0, 0) in component "08_PneumaticSystem (1)"
  line L0 (0, 220, 150) -> (200, 220, 150)
  line L1 (200, 220, 150) -> (200, 300, 150)
  line L2 (200, 300, 150) -> (0, 300, 150)
  line L3 (0, 300, 150) -> (0, 220, 150)
extrude "Extrude3'''''''''''''''" add sketch "Sketch3 (16)" along normal blind 60 separate body contours L0 L1 L2 L3 in plane through (0, 0, 150) normal (0, 0, 1) makes body 185 in component "08_PneumaticSystem (1)"
sketch "Sketch4 (16)" plane through (0, 0, 0) normal (0, 0, 1) x (1, 0, 0) in component "08_PneumaticSystem (1)"
  line L0 (20, 220, 210) -> (60, 220, 210)
  line L1 (60, 220, 210) -> (60, 280, 210)
  line L2 (60, 280, 210) -> (20, 280, 210)
  line L3 (20, 280, 210) -> (20, 220, 210)
extrude "Extrude4'''''''''''''''" add sketch "Sketch4 (16)" along normal blind 40 separate body contours L0 L1 L2 L3 in plane through (0, 0, 210) normal (0, 0, 1) makes body 186 in component "08_PneumaticSystem (1)"
sketch "Sketch5 (14)" plane through (0, 0, 0) normal (0, 0, 1) x (1, 0, 0) in component "08_PneumaticSystem (1)"
  line L0 (80, 220, 210) -> (120, 220, 210)
  line L1 (120, 220, 210) -> (120, 280, 210)
  line L2 (120, 280, 210) -> (80, 280, 210)
  line L3 (80, 280, 210) -> (80, 220, 210)
extrude "Extrude5'''''''''''''" add sketch "Sketch5 (14)" along normal blind 40 separate body contours L0 L1 L2 L3 in plane through (0, 0, 210) normal (0, 0, 1) makes body 187 in component "08_PneumaticSystem (1)"
sketch "Sketch6 (14)" plane through (0, 0, 0) normal (0, 0, 1) x (1, 0, 0) in component "08_PneumaticSystem (1)"
  line L0 (140, 220, 210) -> (180, 220, 210)
  line L1 (180, 220, 210) -> (180, 280, 210)
  line L2 (180, 280, 210) -> (140, 280, 210)
  line L3 (140, 280, 210) -> (140, 220, 210)
extrude "Extrude6'''''''''''''" add sketch "Sketch6 (14)" along normal blind 40 separate body contours L0 L1 L2 L3 in plane through (0, 0, 210) normal (0, 0, 1) makes body 188 in component "08_PneumaticSystem (1)"
sketch "Sketch7 (14)" plane through (0, 0, 0) normal (0, 0, 1) x (1, 0, 0) in component "08_PneumaticSystem (1)"
  circle A0 through (195, 260, 150) (157.5, 281.6506, 150) (157.5, 238.3494, 150)
extrude "Extrude7'''''''''''''" add sketch "Sketch7 (14)" along normal blind 70 separate body contours A0 in plane through (0, 0, 150) normal (0, 0, 1) makes body 189 in component "08_PneumaticSystem (1)"
sketch "Sketch8 (14)" plane through (0, 0, 0) normal (0, 0, 1) x (1, 0, 0) in component "08_PneumaticSystem (1)"
  circle A0 through (50, 260, 150) (20, 277.3205, 150) (20, 242.6795, 150)
extrude "Extrude8'''''''''''''" add sketch "Sketch8 (14)" along normal blind 60 separate body contours A0 in plane through (0, 0, 150) normal (0, 0, 1) makes body 190 in component "08_PneumaticSystem (1)"
sketch "Sketch9 (14)" plane through (0, 0, 0) normal (0, 0, 1) x (1, 0, 0) in component "08_PneumaticSystem (1)"
  line L0 (200, 100, 200) -> (208, 100, 200)
  line L1 (208, 100, 200) -> (208, 250, 200)
  line L2 (208, 250, 200) -> (200, 250, 200)
  line L3 (200, 250, 200) -> (200, 100, 200)
extrude "Extrude9'''''''''''''" add sketch "Sketch9 (14)" along normal blind 8 separate body contours L0 L1 L2 L3 in plane through (0, 0, 200) normal (0, 0, 1) makes body 191 in component "08_PneumaticSystem (1)"
sketch "Sketch10 (14)" plane through (0, 0, 0) normal (0, 0, 1) x (1, 0, 0) in component "08_PneumaticSystem (1)"
  line L0 (230, 100, 200) -> (238, 100, 200)
  line L1 (238, 100, 200) -> (238, 250, 200)
  line L2 (238, 250, 200) -> (230, 250, 200)
  line L3 (230, 250, 200) -> (230, 100, 200)
extrude "Extrude10'''''''''''''" add sketch "Sketch10 (14)" along normal blind 8 separate body contours L0 L1 L2 L3 in plane through (0, 0, 200) normal (0, 0, 1) makes body 192 in component "08_PneumaticSystem (1)"
sketch "Sketch1 (18)" plane through (0, 0, 0) normal (0, 0, 1) x (1, 0, 0) in component "09_TriggerSensor (1)"
  line L0 (780, -50, 100) -> (800, -50, 100)
  line L1 (800, -50, 100) -> (800, -20, 100)
  line L2 (800, -20, 100) -> (780, -20, 100)
  line L3 (780, -20, 100) -> (780, -50, 100)
extrude "Extrude1'''''''''''''''''" add sketch "Sketch1 (18)" along normal blind 150 separate body contours L0 L1 L2 L3 in plane through (0, 0, 100) normal (0, 0, 1) makes body 193 in component "09_TriggerSensor (1)"
sketch "Sketch2 (18)" plane through (0, 0, 0) normal (0, 0, 1) x (1, 0, 0) in component "09_TriggerSensor (1)"
  line L0 (780, -50, 200) -> (800, -50, 200)
  line L1 (800, -50, 200) -> (800, -10, 200)
  line L2 (800, -10, 200) -> (780, -10, 200)
  line L3 (780, -10, 200) -> (780, -50, 200)
extrude "Extrude2'''''''''''''''''" add sketch "Sketch2 (18)" along normal blind 40 separate body contours L0 L1 L2 L3 in plane through (0, 0, 200) normal (0, 0, 1) makes body 194 in component "09_TriggerSensor (1)"
sketch "Sketch1 (19)" plane through (0, 0, 0) normal (0, 0, 1) x (1, 0, 0) in component "01_ConveyorBelt (2)"
  line L0 (50, 0) -> (80, 0)
  line L1 (80, 0) -> (80, 30)
  line L2 (80, 30) -> (50, 30)
  line L3 (50, 30) -> (50, 0)
extrude "Extrude1''''''''''''''''''" add sketch "Sketch1 (19)" along normal blind 100 separate body makes body 195 in component "01_ConveyorBelt (2)"
sketch "Sketch2 (19)" plane through (0, 0, 0) normal (0, 0, 1) x (1, 0, 0) in component "01_ConveyorBelt (2)"
  line L0 (50, 370) -> (80, 370)
  line L1 (80, 370) -> (80, 400)
  line L2 (80, 400) -> (50, 400)
  line L3 (50, 400) -> (50, 370)
extrude "Extrude2''''''''''''''''''" add sketch "Sketch2 (19)" along normal blind 100 separate body makes body 196 in component "01_ConveyorBelt (2)"
sketch "Sketch3 (17)" plane through (0, 0, 0) normal (0, 0, 1) x (1, 0, 0) in component "01_ConveyorBelt (2)"
  line L0 (2950, 0) -> (2980, 0)
  line L1 (2980, 0) -> (2980, 30)
  line L2 (2980, 30) -> (2950, 30)
  line L3 (2950, 30) -> (2950, 0)
extrude "Extrude3''''''''''''''''" add sketch "Sketch3 (17)" along normal blind 100 separate body makes body 197 in component "01_ConveyorBelt (2)"
sketch "Sketch4 (17)" plane through (0, 0, 0) normal (0, 0, 1) x (1, 0, 0) in component "01_ConveyorBelt (2)"
  line L0 (2950, 370) -> (2980, 370)
  line L1 (2980, 370) -> (2980, 400)
  line L2 (2980, 400) -> (2950, 400)
  line L3 (2950, 400) -> (2950, 370)
extrude "Extrude4''''''''''''''''" add sketch "Sketch4 (17)" along normal blind 100 separate body makes body 198 in component "01_ConveyorBelt (2)"
sketch "Sketch5 (15)" plane through (0, 0, 0) normal (0, 0, 1) x (1, 0, 0) in component "01_ConveyorBelt (2)"
  line L0 (0, 0, 100) -> (3000, 0, 100)
  line L1 (3000, 0, 100) -> (3000, 20, 100)
  line L2 (3000, 20, 100) -> (0, 20, 100)
  line L3 (0, 20, 100) -> (0, 0, 100)
extrude "Extrude5''''''''''''''" add sketch "Sketch5 (15)" along normal blind 10 separate body contours L0 L1 L2 L3 in plane through (0, 0, 100) normal (0, 0, 1) makes body 199 in component "01_ConveyorBelt (2)"
sketch "Sketch6 (15)" plane through (0, 0, 0) normal (0, 0, 1) x (1, 0, 0) in component "01_ConveyorBelt (2)"
  line L0 (0, 380, 100) -> (3000, 380, 100)
  line L1 (3000, 380, 100) -> (3000, 400, 100)
  line L2 (3000, 400, 100) -> (0, 400, 100)
  line L3 (0, 400, 100) -> (0, 380, 100)
extrude "Extrude6''''''''''''''" add sketch "Sketch6 (15)" along normal blind 10 separate body contours L0 L1 L2 L3 in plane through (0, 0, 100) normal (0, 0, 1) makes body 200 in component "01_ConveyorBelt (2)"
sketch "Sketch7 (15)" plane through (0, 0, 0) normal (0, 0, 1) x (1, 0, 0) in component "01_ConveyorBelt (2)"
  line L0 (0, 20, 100) -> (3000, 20, 100)
  line L1 (3000, 20, 100) -> (3000, 380, 100)
  line L2 (3000, 380, 100) -> (0, 380, 100)
  line L3 (0, 380, 100) -> (0, 20, 100)
extrude "Extrude7''''''''''''''" add sketch "Sketch7 (15)" along normal blind 10 separate body contours L0 L1 L2 L3 in plane through (0, 0, 100) normal (0, 0, 1) makes body 201 in component "01_ConveyorBelt (2)"
sketch "Sketch8 (15)" plane through (0, 0, 0) normal (0, 0, 1) x (1, 0, 0) in component "01_ConveyorBelt (2)"
  circle A0 through (200, 200, 105) (-55, 347.2243, 105) (-55, 52.7757, 105)
extrude "Extrude8''''''''''''''" add sketch "Sketch8 (15)" along normal blind 30 separate body contours A0 in plane through (0, 0, 105) normal (0, 0, 1) makes body 202 in component "01_ConveyorBelt (2)"
sketch "Sketch9 (15)" plane through (0, 0, 0) normal (0, 0, 1) x (1, 0, 0) in component "01_ConveyorBelt (2)"
  circle A0 through (3140, 200, 105) (2885, 347.2243, 105) (2885, 52.7757, 105)
extrude "Extrude9''''''''''''''" add sketch "Sketch9 (15)" along normal blind 30 separate body contours A0 in plane through (0, 0, 105) normal (0, 0, 1) makes body 203 in component "01_ConveyorBelt (2)"
sketch "Sketch10 (15)" plane through (0, 0, 0) normal (0, 0, 1) x (1, 0, 0) in component "01_ConveyorBelt (2)"
  line L0 (2900, 420, 50) -> (2980, 420, 50)
  line L1 (2980, 420, 50) -> (2980, 500, 50)
  line L2 (2980, 500, 50) -> (2900, 500, 50)
  line L3 (2900, 500, 50) -> (2900, 420, 50)
extrude "Extrude10''''''''''''''" add sketch "Sketch10 (15)" along normal blind 80 separate body contours L0 L1 L2 L3 in plane through (0, 0, 50) normal (0, 0, 1) makes body 204 in component "01_ConveyorBelt (2)"
sketch "Sketch1 (20)" plane through (0, 0, 0) normal (0, 0, 1) x (1, 0, 0) in component "02_VisionStation (2)"
  line L0 (970, -80) -> (1010, -80)
  line L1 (1010, -80) -> (1010, -40)
  line L2 (1010, -40) -> (970, -40)
  line L3 (970, -40) -> (970, -80)
extrude "Extrude1'''''''''''''''''''" add sketch "Sketch1 (20)" along normal blind 600 separate body makes body 205 in component "02_VisionStation (2)"
sketch "Sketch2 (20)" plane through (0, 0, 0) normal (0, 0, 1) x (1, 0, 0) in component "02_VisionStation (2)"
  line L0 (970, 440) -> (1010, 440)
  line L1 (1010, 440) -> (1010, 480)
  line L2 (1010, 480) -> (970, 480)
  line L3 (970, 480) -> (970, 440)
extrude "Extrude2'''''''''''''''''''" add sketch "Sketch2 (20)" along normal blind 600 separate body makes body 206 in component "02_VisionStation (2)"
sketch "Sketch3 (18)" plane through (0, 0, 0) normal (0, 0, 1) x (1, 0, 0) in component "02_VisionStation (2)"
  line L0 (970, -80, 600) -> (1010, -80, 600)
  line L1 (1010, -80, 600) -> (1010, 520, 600)
  line L2 (1010, 520, 600) -> (970, 520, 600)
  line L3 (970, 520, 600) -> (970, -80, 600)
extrude "Extrude3'''''''''''''''''" add sketch "Sketch3 (18)" along normal blind 40 separate body contours L0 L1 L2 L3 in plane through (0, 0, 600) normal (0, 0, 1) makes body 207 in component "02_VisionStation (2)"
sketch "Sketch4 (18)" plane through (0, 0, 0) normal (0, 0, 1) x (1, 0, 0) in component "02_VisionStation (2)"
  line L0 (960, 150, 580) -> (1020, 150, 580)
  line L1 (1020, 150, 580) -> (1020, 250, 580)
  line L2 (1020, 250, 580) -> (960, 250, 580)
  line L3 (960, 250, 580) -> (960, 150, 580)
extrude "Extrude4'''''''''''''''''" add sketch "Sketch4 (18)" along normal blind 20 separate body contours L0 L1 L2 L3 in plane through (0, 0, 580) normal (0, 0, 1) makes body 208 in component "02_VisionStation (2)"
sketch "Sketch5 (16)" plane through (0, 0, 0) normal (0, 0, 1) x (1, 0, 0) in component "02_VisionStation (2)"
  line L0 (965, 160, 540) -> (1015, 160, 540)
  line L1 (1015, 160, 540) -> (1015, 240, 540)
  line L2 (1015, 240, 540) -> (965, 240, 540)
  line L3 (965, 240, 540) -> (965, 160, 540)
extrude "Extrude5'''''''''''''''" add sketch "Sketch5 (16)" along normal blind 40 separate body contours L0 L1 L2 L3 in plane through (0, 0, 540) normal (0, 0, 1) makes body 209 in component "02_VisionStation (2)"
sketch "Sketch6 (16)" plane through (0, 0, 0) normal (0, 0, 1) x (1, 0, 0) in component "02_VisionStation (2)"
  circle A0 through (1002, 200, 520) (984, 210.3923, 520) (984, 189.6077, 520)
extrude "Extrude6'''''''''''''''" add sketch "Sketch6 (16)" along normal blind 20 separate body contours A0 in plane through (0, 0, 520) normal (0, 0, 1) makes body 210 in component "02_VisionStation (2)"
sketch "Sketch7 (16)" plane through (0, 0, 0) normal (0, 0, 1) x (1, 0, 0) in component "02_VisionStation (2)"
  line L0 (940, 180, 490) -> (1040, 180, 490)
  line L1 (1040, 180, 490) -> (1040, 220, 490)
  line L2 (1040, 220, 490) -> (940, 220, 490)
  line L3 (940, 220, 490) -> (940, 180, 490)
extrude "Extrude7'''''''''''''''" add sketch "Sketch7 (16)" along normal blind 25 separate body contours L0 L1 L2 L3 in plane through (0, 0, 490) normal (0, 0, 1) makes body 211 in component "02_VisionStation (2)"
sketch "Sketch8 (16)" plane through (0, 0, 0) normal (0, 0, 1) x (1, 0, 0) in component "02_VisionStation (2)"
  circle A0 through (972, 195, 480) (961.5, 201.0622, 480) (961.5, 188.9378, 480)
extrude "Extrude8'''''''''''''''" add sketch "Sketch8 (16)" along normal blind 10 separate body contours A0 in plane through (0, 0, 480) normal (0, 0, 1) makes body 212 in component "02_VisionStation (2)"
sketch "Sketch9 (16)" plane through (0, 0, 0) normal (0, 0, 1) x (1, 0, 0) in component "02_VisionStation (2)"
  circle A0 through (1022, 195, 480) (1011.5, 201.0622, 480) (1011.5, 188.9378, 480)
extrude "Extrude9'''''''''''''''" add sketch "Sketch9 (16)" along normal blind 10 separate body contours A0 in plane through (0, 0, 480) normal (0, 0, 1) makes body 213 in component "02_VisionStation (2)"
sketch "Sketch10 (16)" plane through (0, 0, 0) normal (0, 0, 1) x (1, 0, 0) in component "02_VisionStation (2)"
  circle A0 through (1025, 200, 530) (972.5, 230.3109, 530) (972.5, 169.6891, 530)
extrude "Extrude10'''''''''''''''" add sketch "Sketch10 (16)" along normal blind 5 separate body contours A0 in plane through (0, 0, 530) normal (0, 0, 1) makes body 214 in component "02_VisionStation (2)"
sketch "Sketch1 (21)" plane through (0, 0, 0) normal (0, 0, 1) x (1, 0, 0) in component "03_RobotBase (2)"
  line L0 (-200, -200) -> (200, -200)
  line L1 (200, -200) -> (200, 200)
  line L2 (200, 200) -> (-200, 200)
  line L3 (-200, 200) -> (-200, -200)
extrude "Extrude1''''''''''''''''''''" add sketch "Sketch1 (21)" along normal blind 30 separate body makes body 215 in component "03_RobotBase (2)"
sketch "Sketch2 (21)" plane through (0, 0, 0) normal (0, 0, 1) x (1, 0, 0) in component "03_RobotBase (2)"
  circle A0 through (150, 0, 30) (-75, 129.9038, 30) (-75, -129.9038, 30)
extrude "Extrude2''''''''''''''''''''" add sketch "Sketch2 (21)" along normal blind 100 separate body contours A0 in plane through (0, 0, 30) normal (0, 0, 1) makes body 216 in component "03_RobotBase (2)"
sketch "Sketch3 (19)" plane through (0, 0, 0) normal (0, 0, 1) x (1, 0, 0) in component "03_RobotBase (2)"
  circle A0 through (120, 0, 130) (-60, 103.923, 130) (-60, -103.923, 130)
extrude "Extrude3''''''''''''''''''" add sketch "Sketch3 (19)" along normal blind 20 separate body contours A0 in plane through (0, 0, 130) normal (0, 0, 1) makes body 217 in component "03_RobotBase (2)"
sketch "Sketch4 (19)" plane through (0, 0, 0) normal (0, 0, 1) x (1, 0, 0) in component "03_RobotBase (2)"
  line L0 (80, -40, 50) -> (136, -40, 50)
  line L1 (136, -40, 50) -> (136, 16, 50)
  line L2 (136, 16, 50) -> (80, 16, 50)
  line L3 (80, 16, 50) -> (80, -40, 50)
extrude "Extrude4''''''''''''''''''" add sketch "Sketch4 (19)" along normal blind 76 separate body contours L0 L1 L2 L3 in plane through (0, 0, 50) normal (0, 0, 1) makes body 218 in component "03_RobotBase (2)"
sketch "Sketch1 (22)" plane through (0, 0, 0) normal (0, 0, 1) x (1, 0, 0) in component "04_RobotArm (2)"
  circle A0 through (80, 0, 150) (-40, 69.282, 150) (-40, -69.282, 150)
extrude "Extrude1'''''''''''''''''''''" add sketch "Sketch1 (22)" along normal blind 40 separate body contours A0 in plane through (0, 0, 150) normal (0, 0, 1) makes body 219 in component "04_RobotArm (2)"